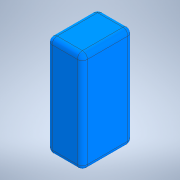
# Autodesk Inventor part: battery
Saved by Autodesk Inventor 2022.6 (Build 266554000, 554)
## iProperties
Created: 2024-10-06
Part Number: battery
Material: Genérico
Document SubType Name: Modeling
Designer: Olá
Density: 1 g/cm^3
Appearance: Padrão
Author: Olá
Autodesk Inventor part; units mm, degrees
ref_plane "YZ Plane" through (0, 0, 0) normal (1, 0, 0) x (0, 1, 0)
ref_plane "XZ Plane" through (0, 0, 0) normal (0, 1, 0) x (-1, 0, 0)
ref_plane "XY Plane" through (0, 0, 0) normal (0, 0, 1) x (1, 0, 0)
sketch "Esboço1" plane through (0, 0, 0) normal (1, 0, 0) x (0, 1, 0)
  line L0 (0, 0) -> (200, 0)
  line L1 (200, 0) -> (200, -100)
  line L2 (200, -100) -> (0, -100)
  line L3 (0, -100) -> (0, 0)
  dimension "d0" = 200
  dimension "d1" = 100
  constraints: 8 end point, 2 parallel, 1 horizontal, 1 perpendicular
  measures "d0" distance of L1.end L2.end
  measures "d1" distance of L0.end L1.end
extrude "Extrusão1" add sketch "Esboço1" along normal blind 70
fillet "Arredondamento1" radius 10 12 edges at (35, 200, 0) (70, 200, -50) (0, 200, -50) (35, 200, -100) (35, 0, 0) (70, 0, -50) (0, 0, -50) (35, 0, -100) (70, 100, 0) (0, 100, 0) (70, 100, -100) (0, 100, -100)
